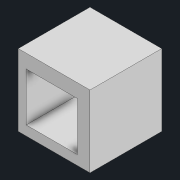
# Autodesk Inventor part: Zohair did a thing
Saved by Autodesk Inventor 2022 (Build 260153000, 153)
## iProperties
Created: 2021-09-17
Part Number: Zohair did a thing
Material: Generic
Document SubType Name: Modeling
Designer: divid
Density: 1 g/cm^3
Appearance: Default
Author: divid
Autodesk Inventor part; units mm, degrees
ref_plane "YZ Plane" through (0, 0, 0) normal (1, 0, 0) x (0, 1, 0)
ref_plane "XZ Plane" through (0, 0, 0) normal (0, 1, 0) x (-1, 0, 0)
ref_plane "XY Plane" through (0, 0, 0) normal (0, 0, 1) x (1, 0, 0)
sketch "Sketch1" plane through (0, 0, 0) normal (0, 1, 0) x (-1, 0, 0)
  line L0 (13.0479, 11.7432) -> (-12.3521, 11.7432)
  line L1 (-12.3521, 11.7432) -> (-12.3521, -13.6568)
  line L2 (-12.3521, -13.6568) -> (13.0479, -13.6568)
  line L3 (13.0479, -13.6568) -> (13.0479, 11.7432)
  point P0 (0, 0)
  dimension "d0" = 25.4
  dimension "d1" = 25.4
  constraints: 8 end point, 2 parallel, 1 horizontal, 1 perpendicular
  measures "d0" distance of L1.end L2.end
  measures "d1" distance of L0.end L1.end
extrude "Extrusion1" add sketch "Sketch1" along normal blind 25.4
sketch "Sketch2" plane through (-13.0479, 0, 11.7432) normal (0, 0, 1) x (1, 0, 0)
  line L0 (2.8121, 3.3867) -> (20.955, 3.3867)
  line L1 (20.955, 3.3867) -> (20.955, 20.5619)
  line L2 (20.955, 20.5619) -> (2.8121, 20.5619)
  line L3 (2.8121, 20.5619) -> (2.8121, 3.3867)
  point P0 (13.0479, 0)
  constraints: 8 end point, 2 parallel, 1 horizontal, 1 perpendicular
extrude "Extrusion2" cut sketch "Sketch2" against normal blind 25.4
body "Solid1"
